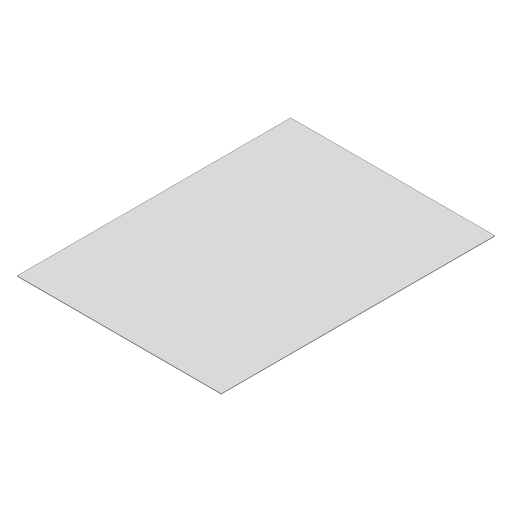
# Autodesk Inventor part: Base_Plate
Saved by Autodesk Inventor 2024.2 (Build 282272000, 272)
## iProperties
Created: 2025-01-06
Part Number: Base_Plate
Material: Generic
Document SubType Name: Modeling
Designer: Kartik
Mass: 544.752 g
Surface Area: 9111.89 cm^2
Volume: 544.752 cm^3
Density: 1 g/cm^3
Appearance: Default
Author: Kartik
Autodesk Inventor part; units mm, degrees
ref_plane "YZ Plane" through (0, 0, 0) normal (1, 0, 0) x (0, 1, 0)
ref_plane "XZ Plane" through (0, 0, 0) normal (0, 1, 0) x (-1, 0, 0)
ref_plane "XY Plane" through (0, 0, 0) normal (0, 0, 1) x (1, 0, 0)
sketch "Sketch1" plane through (0, 0, 0) normal (0, 1, 0) x (-1, 0, 0)
  line L0 (291, 390) -> (-291, 390)
  line L1 (-291, 390) -> (-291, -390)
  line L2 (-291, -390) -> (291, -390)
  line L3 (291, -390) -> (291, 390)
  point P0 (0, 0)
  dimension "d0" = 780
  dimension "d1" = 390
  dimension "d2" = 582
  dimension "d3" = 291
  constraints: 8 end point, 2 parallel, 1 horizontal, 1 perpendicular
  measures "d0" distance of L2.end L0.start
  measures "d1" distance from line of L2 point (0, 0)
  measures "d2" distance of L0.start L0.end
  measures "d3" distance from line of L1 point (0, 0)
extrude "Extrusion1" add sketch "Sketch1" along normal blind 1.2
equation "\"d1\" = 0.5 * d0"
equation "\"d3\" = 0.5 * d2"
body "Solid1"
